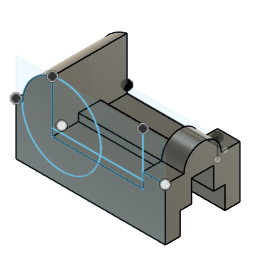
Robocon Task1 Image 2 v1 (Autodesk Fusion 360 design; units mm, degrees)
Autodesk Fusion 360 part; units mm, degrees
note: some values were not read from the file. Set by a fixed rule: which sketch regions a step uses.
sketch "Sketch1" plane through (0, 0, 0) normal (0, 0, 1) x (1, 0, 0)
  line L0 (50, -25) -> (-50, -25)
  line L1 (-50, -25) -> (-50, 25)
  line L2 (-50, 25) -> (50, 25)
  line L3 (50, 25) -> (50, -25)
  line L4 (50, -25) -> (-50, 25) construction
  line L5 (-50, -25) -> (50, 25) construction
  dimension "d1" = 100
  dimension "d2" = 50
  constraint horizontal L0
  constraint perpendicular L0 L1
  constraint parallel L0 L2
  constraint parallel L1 L3
  constraint coincident L4 origin
  constraint coincident L5 origin
  measures "d1" distance of L1.end L2.end
  measures "d2" distance of L0.end L1.end
extrude "Extrude1" add sketch "Sketch1" along normal blind 60
sketch "Sketch2" plane through (0, -25, 0) normal (0, -1, 0) x (1, 0, 0)
  line L0 (-50, 0) -> (50, 0)
  line L1 (50, 0) -> (50, 60)
  line L2 (50, 60) -> (-50, 60)
  line L3 (-50, 60) -> (-50, 0)
  line L4 (-50, 35.014) -> (-45.6262, 35.014)
  circle A0 centre (-19.3951, 34.5262) radius 26.2357
  line L5 (-25.6715, 60) -> (-25.6715, 25.0092)
  line L6 (-25.6715, 25.0092) -> (35, 25.0092)
  line L7 (35, 25.0092) -> (35, 60)
  line L8 (35, 30.0471) -> (-25.6715, 30.0471)
  line L9 (35, 30.0471) -> (35, 35.0471)
  line L10 (35, 35.0471) -> (50, 35.0471)
  dimension "d25" = 5
  constraint coincident L3 L4.start
  constraint perpendicular L3 L4
  constraint coincident L4.end A0
  constraint coincident A0 L5.start
  constraint coincident L2 L5.start
  constraint perpendicular L0 L5
  constraint perpendicular L5 L6
  constraint coincident L2 L7.end
  constraint perpendicular L2 L7
  constraint coincident L7 L8.start
  constraint coincident L5 L8.end
  constraint perpendicular L5 L8
  constraint perpendicular L8 L9
  constraint perpendicular L7 L10
  measures "d25" distance of L8.start L9.end
extrude "Extrude2" cut sketch "Sketch2" against normal blind 100 contours L2 A0 L7 L8 L9
extrude "Extrude3" cut sketch "Sketch2" against normal blind 100 contours L2 A0 | L2 A0 L5 L8
extrude "Extrude4" cut sketch "Sketch2" against normal blind 17.5 contours A0 L5 L6 L8 | A0 L6 L7 L8
extrude "Extrude5" cut sketch "Sketch2" against normal blind 100 contours L2 L3 L4 A0
sketch "Sketch3" plane through (-50, 0, 0) normal (-1, 0, 0) x (0, -1, 0)
  line L0 (25, 35.014) -> (-25, 35.014)
  line L1 (-25, 35.014) -> (-25, 0)
  line L2 (-25, 0) -> (25, 0)
  line L3 (25, 0) -> (25, 35.014)
  line L4 (-25, 0) -> (-15, 0)
  line L5 (25, 0) -> (15, 0)
  line L6 (15, 0) -> (15, 15)
  line L7 (-15, 0) -> (-15, 15)
  line L8 (-7.4, 15) -> (-7.4, 30)
  line L9 (7.4, 15) -> (7.4, 30)
  line L10 (7.4, 30) -> (-7.4, 30)
  line L11 (-15, 15) -> (-7.4, 15)
  line L12 (15, 15) -> (7.4, 15)
  dimension "d21" = 7.6
  dimension "d22" = 7.6
  constraint coincident L1.end L2.start
  constraint perpendicular L1 L4
  constraint coincident L2.end L3.start
  constraint perpendicular L3 L5
  constraint perpendicular L5 L6
  constraint perpendicular L4 L7
  constraint perpendicular L8 L10
  constraint perpendicular L7 L11
  constraint perpendicular L9 L12
  measures "d21" distance of L7.end L8.start
  measures "d22" distance of L6.end L9.start
extrude "Extrude6" cut sketch "Sketch3" against normal blind 100 contours L2 L6 L7 L8 L9 L10 L11 L12
extrude "Extrude7" cut sketch "Sketch2" against normal blind 2 contours L1 L2 L7 L10
sketch "Sketch4" plane through (50, 0, 0) normal (1, 0, 0) x (0, 1, 0)
  line L0 (-23, 35.0471) -> (-25, 35.0471)
  line L1 (-25, 35.0471) -> (-25, 0)
  line L2 (-25, 0) -> (-15, 0)
  line L3 (-15, 0) -> (-15, 15)
  line L4 (-15, 15) -> (-7.4, 15)
  line L5 (-7.4, 15) -> (-7.4, 30)
  line L6 (-7.4, 30) -> (7.4, 30)
  line L7 (7.4, 30) -> (7.4, 15)
  line L8 (7.4, 15) -> (15, 15)
  line L9 (15, 15) -> (15, 0)
  line L10 (15, 0) -> (25, 0)
  line L11 (25, 0) -> (25, 60)
  line L12 (25, 60) -> (-23, 60)
  line L13 (-23, 60) -> (-23, 35.0471)
  line L14 (-25, 35.0471) -> (25, 35.0471)
  circle A0 centre (0, 35.0471) radius 12.5
  dimension "d28" = 25
  constraint coincident L0.end L1.start
  constraint coincident L11 L14.end
  constraint perpendicular L11 L14
  constraint midpoint L14 A0.centre
  measures "d28" diameter of A0
extrude "Extrude8" cut sketch "Sketch4" against normal blind 50 contours L11 L12 L13 L14 A0
sketch "Sketch5" plane through (0, 25, 0) normal (0, 1, 0) x (-1, 0, 0)
  line L0 (-35, 35.0471) -> (-50, 35.0471)
  line L1 (-50, 35.0471) -> (-50, 0)
  line L2 (-50, 0) -> (50, 0)
  line L3 (50, 0) -> (50, 35.014)
  line L4 (50, 35.014) -> (45.6262, 35.014)
  arc A0 (45.6262, 35.014) -> (25.6715, 60) centre (19.3951, 34.5262) ccw
  line L5 (25.6715, 60) -> (25.6715, 30.0471)
  line L6 (25.6715, 30.0471) -> (-35, 30.0471)
  line L7 (-35, 30.0471) -> (-35, 35.0471)
  line L8 (25.6715, 30.0471) -> (25.6715, 25.0471)
  line L9 (25.6715, 25.0471) -> (-29.3285, 25.0471)
  line L10 (-29.3285, 25.0471) -> (-35, 30.0471)
  line L11 (-35, 30.0471) -> (-35, 17)
  line L12 (-29.3285, 25.0471) -> (-40, 25.0471)
  dimension "d31" = 5
  dimension "d32" = 55
  constraint coincident L5.end L6.start
  constraint perpendicular L6 L8
  constraint perpendicular L8 L9
  constraint coincident L6.end L7.start
  constraint perpendicular L6 L11
  constraint perpendicular L11 L12
  measures "d31" distance of L5.end L8.end
  measures "d32" distance of L8.end L9.end
extrude "Extrude9" cut sketch "Sketch5" against normal blind 17.5 contours L6 L8 L9 L10
extrude "Extrude10" cut sketch "Sketch5" against normal blind 17.5 contours L10 L11 L12
